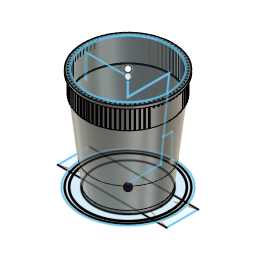
2023_05_26_SobaSTL v3 (Autodesk Fusion 360 design; units mm, degrees)
Autodesk Fusion 360 part; units mm, degrees
sketch "Sketch2" plane through (0, 0, 0) normal (0, 0, 1) x (1, 0, 0)
  circle A0 centre (0, 0) radius 34.65
  circle A1 centre (0, 0) radius 34
  dimension "d5" = 69.3
  dimension "d6" = 68
  constraint coincident A0.centre A1.centre
  constraint concentric A0 A1
  measures "d5" diameter of A0
  measures "d6" diameter of A1
extrude "Extrude2" add sketch "Sketch2" along normal blind 2.4 makes body 1
extrude "Extrude3" add sketch "Sketch2" along normal blind 1 separate body contours A0 | A1 makes body 2
move_body "Move1" bodies 2 to x (1, 0, 0) y (0, 1, 0) z (0, 0, 1) at (0, 0, 2.4)
sketch "Sketch3" plane through (0, 0, 0) normal (0, 0, 1) x (1, 0, 0)
  circle A0 centre (0, 0) radius 47.07
  circle A1 centre (0, 0) radius 43.5
  circle A2 centre (0, 0) radius 46.57
  dimension "d11" = 94.14
  dimension "d12" = 87
  dimension "d13" = -0.5
  constraint coincident A0.centre A1.centre
  constraint concentric A0 A1
  measures "d11" diameter of A0
  measures "d12" diameter of A1
extrude "Extrude4" add sketch "Sketch3" along normal blind 3.22 separate body contours A0 | A2 makes body 3
extrude "Extrude5" cut sketch "Sketch3" along normal blind 2.85 contours A1 | A2 bodies 3
move_body "Move2" bodies 3 to x (1, 0, 0) y (0, 1, 0) z (0, 0, 1) at (0, 0, -3.22)
move_body "Move3" bodies 3 to x (1, 0, 0) y (0, 1, 0) z (0, 0, 1) at (0, 0, 107)
sketch "Sketch4" plane through (0, 0, 0) normal (0, 0, 1) x (1, 0, 0)
  circle A0 centre (0, 0) radius 43.5
  dimension "d22" = 87
  constraint coincident A0.centre origin
  measures "d22" diameter of A0
sketch "Sketch5" plane through (0, 0, 0) normal (0, 1, 0) x (1, 0, 0)
  line L0 (0, -100) -> (-43.5, -100)
  line L1 (-43.5, -100) -> (-45, -100)
  line L2 (-45, -100) -> (-45, -75.25)
  line L3 (-45, -75.25) -> (-43.5, -75.25)
  line L4 (-43.5, -75.25) -> (-43.5, -100)
  line L5 (-43.5, -75.25) -> (-43.5, -77)
  line L6 (-43.5, -77) -> (-45, -77)
  line L7 (-45, -77) -> (-43.5, -75.25)
  dimension "d23" = 43.5
  dimension "d24" = 1.5
  dimension "d25" = 24.75
  dimension "d26" = 1.75
  constraint horizontal L0
  constraint horizontal L1
  constraint vertical L2
  constraint horizontal L3
  constraint vertical L4
  constraint perpendicular L3 L5
  constraint coincident L2 L6.end
  constraint perpendicular L4 L6
  measures "d23" distance of L0.start L0.end
  measures "d24" distance of L0.end L1.end
  measures "d25" distance of L0.end L3.end
  measures "d26" distance of L3.end L5.end
extrude "Extrude6" add sketch "Sketch5" along normal blind 0.77 separate body contours L1 L2 L4 L6 | L4 L5 L6 L7 makes body 4
pattern_circular "C-Pattern1" count 76 over 360 about axis through (0, 0, 107) along (0, 0, -1) of bodies 4 makes body 5 at (-44.348, 3.6748, 84.6667) makes body 6 at (-43.3999, 7.2422, 84.6667) makes body 7 at (-42.6536, 10.8014, 84.6667) makes body 8 at (-41.616, 14.2868, 84.6667) makes body 9 at (-40.294, 17.6746, 84.6667) makes body 10 at (-38.6968, 20.9417, 84.6667) makes body 11 at (-36.8353, 24.0657, 84.6667) makes body 12 at (-34.7222, 27.0254, 84.6667) makes body 13 at (-32.3719, 29.8004, 84.6667) makes body 14 at (-29.8004, 32.3719, 84.6667) makes body 15 at (-27.0254, 34.7222, 84.6667) makes body 16 at (-24.3392, 37.2539, 84.6667) makes body 17 at (-20.9417, 38.6968, 84.6667) makes body 18 at (-17.6746, 40.294, 84.6667) makes body 19 at (-14.2868, 41.616, 84.6667) makes body 20 at (-10.8014, 42.6536, 84.6667) makes body 21 at (-7.3245, 43.8931, 84.6667) makes body 22 at (-3.6335, 43.8497, 84.6667) makes body 23 at (0, 44.5, 84.6667) makes body 24 at (3.6748, 44.348, 84.6667) makes body 25 at (7.2422, 43.3999, 84.6667) makes body 26 at (10.8014, 42.6536, 84.6667) makes body 27 at (14.2868, 41.616, 84.6667) makes body 28 at (17.6746, 40.294, 84.6667) makes body 29 at (20.9417, 38.6968, 84.6667) makes body 30 at (24.0657, 36.8353, 84.6667) makes body 31 at (27.0254, 34.7222, 84.6667) makes body 32 at (30.139, 32.7397, 84.6667) makes body 33 at (32.3719, 29.8004, 84.6667) makes body 34 at (34.7222, 27.0254, 84.6667) makes body 35 at (36.8353, 24.0657, 84.6667) makes body 36 at (38.6968, 20.9417, 84.6667) makes body 37 at (40.294, 17.6746, 84.6667) makes body 38 at (41.616, 14.2868, 84.6667) makes body 39 at (42.6536, 10.8014, 84.6667) makes body 40 at (43.3999, 7.2422, 84.6667) makes body 41 at (44.348, 3.6748, 84.6667) makes body 42 at (44.5, 0, 84.6667) makes body 43 at (44.348, -3.6748, 84.6667) makes body 44 at (43.3999, -7.2422, 84.6667) makes body 45 at (42.6536, -10.8014, 84.6667) makes body 46 at (42.0889, -14.4491, 84.6667) makes body 47 at (40.294, -17.6746, 84.6667) makes body 48 at (38.6968, -20.9417, 84.6667) makes body 49 at (37.2539, -24.3392, 84.6667) makes body 50 at (35.1168, -27.3325, 84.6667) makes body 51 at (32.7397, -30.139, 84.6667) makes body 52 at (29.8004, -32.3719, 84.6667) makes body 53 at (27.0254, -34.7222, 84.6667) makes body 54 at (23.4211, -37.2565, 84.6667) makes body 55 at (20.9417, -38.6968, 84.6667) makes body 56 at (17.6746, -40.294, 84.6667) makes body 57 at (14.2868, -41.616, 84.6667) makes body 58 at (10.8014, -42.6536, 84.6667) makes body 59 at (7.3245, -43.8931, 84.6667) makes body 60 at (3.6335, -43.8497, 84.6667) makes body 61 at (0, -44.5, 84.6667) makes body 62 at (-4.4422, -44.2844, 84.6667) makes body 63 at (-7.2422, -43.3999, 84.6667) makes body 64 at (-10.8014, -42.6536, 84.6667) makes body 65 at (-14.4491, -42.0889, 84.6667) makes body 66 at (-17.6746, -40.294, 84.6667) makes body 67 at (-20.9417, -38.6968, 84.6667) makes body 68 at (-24.3392, -37.2539, 84.6667) makes body 69 at (-27.0254, -34.7222, 84.6667) makes body 70 at (-29.8004, -32.3719, 84.6667) makes body 71 at (-32.3719, -29.8004, 84.6667) makes body 72 at (-34.7222, -27.0254, 84.6667) makes body 73 at (-36.8353, -24.0657, 84.6667) makes body 74 at (-38.6968, -20.9417, 84.6667) makes body 75 at (-40.7519, -17.8754, 84.6667) makes body 76 at (-41.616, -14.2868, 84.6667) makes body 77 at (-42.6536, -10.8014, 84.6667) makes body 78 at (-43.3999, -7.2422, 84.6667) makes body 79 at (-43.8497, -3.6335, 84.6667)
move_body "Move4" bodies 4 66 9 60 62 67 63 79 34 73 23 16 52 65 42 17 8 11 26 57 27 45 19 68 38 15 53 50 72 59 10 12 7 75 64 5 77 30 54 55 29 31 74 70 69 61 24 37 44 13 56 39 78 58 71 20 40 51 6 14 33 25 22 76 36 21 47 32 41 28 48 18 46 35 43 49 to x (1, 0, 0) y (0, 1, 0) z (0, 0, 1) at (0, 0, 7)
sketch "Sketch6" plane through (0, 0, 107) normal (0, 0, 1) x (-1, 0, 0)
  circle A0 centre (0, 0) radius 43.5
  circle A1 centre (0, 0) radius 47.07
  circle A2 centre (0, 0) radius 43.5
  circle A3 centre (0, 0) radius 43
  circle A4 centre (0, 0) radius 42.6
  dimension "d34" = 87
  dimension "d35" = -0.5
  dimension "d38" = -0.9
  measures "d34" diameter of A2
extrude "Extrude7" add sketch "Sketch6" against normal blind 23.2 contours A0 A2 bodies 3 4 5 6 7 8 9 10 11 12 13 14 15 16 17 18 19 20 21 22 23 24 25 26 27 28 29 30 31 32 33 34 35 36 37 38 39 40 41 42 43 44 45 46 47 48 49 50 51 52 53 54 55 56 57 58 59 60 61 62 63 64 65 66 67 68 69 70 71 72 73 74 75 76 77 78 79
extrude "Extrude8" add sketch "Sketch6" along normal blind 1 separate body contours A0 A2 | A3 makes body 80
move_body "Move5" bodies 80 to x (1, 0, 0) y (0, 1, 0) z (0, 0, 1) at (0, 0, -24.2)
extrude "Extrude9" add 1 faces at (37.314, 21.5433, 83.8) along direction (0, 0, -1) blind 2 on bodies 3 bodies 3
extrude "Extrude10" add sketch "Sketch6" along normal blind 1 separate body contours A0 A2 | A3 | A4 makes body 81
sketch "Sketch7" plane through (0, 0, 0) normal (1, 0, 0) x (0, 1, 0)
  line L0 (0, 0) -> (0, 3.4)
  line L1 (0, 3.4) -> (34.65, 3.4)
  line L2 (0, 107) -> (0, 81.7874)
  line L3 (0, 81.7874) -> (43.5, 81.7874)
  line L4 (34.65, 3.4) -> (43.5, 81.7874)
  line L5 (-0.5, 0) -> (-0.5, 3.9)
  line L6 (-0.5, 3.9) -> (34.2033, 3.9)
  line L7 (34.2033, 3.9) -> (42.9404, 81.2874)
  line L8 (-0.5, 81.2874) -> (42.9404, 81.2874)
  line L9 (-0.5, 107) -> (-0.5, 81.2874)
  line L10 (42.9404, 81.2874) -> (42.9968, 81.7874)
  line L11 (34.2033, 3.9) -> (34.1468, 3.4)
  line L12 (46, 0) -> (46, 27)
  line L13 (46, 27) -> (36.4318, 27)
  line L14 (36.4318, 27) -> (36.4318, 27.4333)
  line L15 (36.4318, 27.4333) -> (46, 27.4333)
  line L16 (46, 27.4333) -> (46, 27)
  line L17 (42.6691, 81.2874) -> (42.6691, 81.7874)
  dimension "d45" = 34.65
  dimension "d46" = 43.5
  dimension "d47" = -0.5
  dimension "d57" = 27
  constraint coincident L0.start origin
  constraint vertical L0
  constraint perpendicular L0 L1
  constraint vertical L2
  constraint perpendicular L2 L3
  constraint coincident L3 L10.end
  constraint parallel L7 L10
  constraint coincident L1 L11.end
  constraint parallel L7 L11
  constraint vertical L12
  constraint perpendicular L12 L13
  constraint perpendicular L13 L14
  constraint perpendicular L14 L15
  constraint perpendicular L13 L16
  constraint coincident L8 L17.start
  constraint coincident L3 L17.end
  constraint perpendicular L3 L17
  measures "d45" distance of L0.end L1.end
  measures "d46" distance of L2.end L3.end
  measures "d57" distance of L12.start L12.end
revolve "Revolve1" add sketch "Sketch7" angle 360 about axis through (0, 0, 1.75) along (0, 0, 1) contours L1 L4 L7 L11 L13 | L4 L7 L13 L15 | L7 L13 L14 L15 | L3 L4 L7 L10 L15 | L3 L8 L10 L17 bodies 2
delete_body "RemoveBody1" bodies 81
extrude "Extrude11" add 1 faces at (-45, 0.2567, 99.0867) along direction (-1, 0, 0) blind 0.189 on bodies 3 bodies 3
sketch "Sketch8" plane through (0, 0, 0) normal (0, 0, 1) x (1, 0, 0)
  circle A0 centre (0, 0) radius 43.5
  circle A1 centre (0, 0) radius 43.5
  line L0 (56.7613, 16.5) -> (-56.7613, 16.5)
  line L1 (-56.7613, 16.5) -> (-56.7613, -16.5)
  line L2 (-56.7613, -16.5) -> (56.7613, -16.5)
  line L3 (56.7613, -16.5) -> (56.7613, 16.5)
  line L4 (56.7613, 16.5) -> (-56.7613, -16.5) construction
  line L5 (-56.7613, 16.5) -> (56.7613, -16.5) construction
  circle A2 centre (0, 0) radius 49.163
  dimension "d51" = 87
  dimension "d52" = 87
  dimension "d53" = 33
  constraint coincident A0.centre A1.centre
  constraint concentric A0 A1
  constraint horizontal L0
  constraint perpendicular L0 L1
  constraint parallel L0 L2
  constraint parallel L1 L3
  constraint coincident L4 A0.centre
  constraint coincident L5 A0.centre
  constraint concentric A0 A2
  measures "d51" diameter of A0
  measures "d52" diameter of A1
  measures "d53" distance of L0.end L1.end
extrude "Extrude12" cut sketch "Sketch8" along normal blind 100 contours A0 A1 L0 L2 A2 | A0 A1 L0 L2 A2 | L0 L2 L3 A2 | L0 L1 L2 A2 bodies 3
chamfer "Chamfer1" distance 0.74 angle 45 19 edges at (-43.5285, 11.4201, 100) (-44.3229, 7.7865, 100) (-44.0353, 4.4215, 100) (-45.189, 0.385, 100) (-44.4496, -7.027, 100) (-44.8781, -3.3324, 100) (-43.7175, -10.6736, 100) (-42.6868, -14.2473, 100) (-44.8145, 4.0998, 100) (-42.4368, 14.9756, 100) (42.6868, 14.2473, 100) (43.7175, 10.6736, 100) (44.4496, 7.027, 100) (44.8781, 3.3324, 100) (45, -0.385, 100) (44.8145, -4.0998, 100) (44.3229, -7.7865, 100) (43.5285, -11.4201, 100) (42.4368, -14.9756, 100) on bodies 3
combine "Combine1" operation add target body 2 tool bodies 3 1 makes body 82 at (-42.9465, 2.1434, 90.2)
combine "Combine2" operation add target body 82 tool bodies 2 makes body 83 at (39.12, -15.3535, 68.7228)
extrude "Extrude13" add 1 faces at (-4.2809, -42.9022, 81.7874) along direction (0, 0, 1) blind 0.2 on bodies 83 bodies 83 82
fillet "Fillet1" radius 0.3 1 edges at (-43.8846, -17.0212, 107) on bodies 83
hidden bodies 80
equation "d23 = ( 87 / 2 ) * 1 mm"
equation "d45 = ( 69.3 / 2 ) * 1 mm"
equation "d46 = ( 87 / 2 ) * 1 mm"
equation "d57 = 107 mm - 80 mm"
